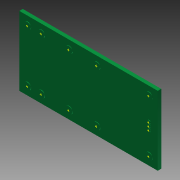
# Autodesk Inventor part: PDU
Saved by Autodesk Inventor 2011 SP1 (Build 150282100, 282)
## iProperties
Created: 2011-06-14
Part Number: PDU
Document SubType Name: Modeling
Designer: Andrew G. Meyer
Mass: 3.22222 g
Surface Area: 43.638 cm^2
Volume: 3.22222 cm^3
Density: 1 g/cm^3
GlobalPropertyList: <PropertyList/>
Author: Andrew G. Meyer
Autodesk Inventor part; units mm, degrees
ref_plane "YZ Plane" through (0, 0, 0) normal (1, 0, 0) x (0, 1, 0)
ref_plane "XZ Plane" through (0, 0, 0) normal (0, 1, 0) x (-1, 0, 0)
ref_plane "XY Plane" through (0, 0, 0) normal (0, 0, 1) x (1, 0, 0)
sketch "Sketch1" plane through (0, 0, 0) normal (0, 0, 1) x (1, 0, 0)
  line L0 (-25.8084, 16.7799) -> (37.6916, 16.7799)
  line L1 (37.6916, 16.7799) -> (37.6916, -14.9701)
  line L2 (37.6916, -14.9701) -> (-25.8084, -14.9701)
  line L3 (-25.8084, -14.9701) -> (-25.8084, 16.7799)
  point P0 (0, 0)
  dimension "d0" = 31.75
  dimension "d1" = 63.5
  constraints: 8 end point, 2 parallel, 1 horizontal, 1 perpendicular
  measures "d0" distance of L2.end L0.start
  measures "d1" distance of L0.start L0.end
extrude "Extrusion1" add sketch "Sketch1" along normal blind 1.5875
sketch "Sketch2" plane through (0, 0, 1.5875) normal (0, 0, 1) x (1, 0, 0)
  line L0 (37.6916, 16.7799) -> (37.6916, -14.9701) projected
  line L1 (-25.8084, 16.7799) -> (37.6916, 16.7799) projected
  line L2 (-25.8084, -14.9701) -> (-25.8084, 16.7799) projected
  line L3 (37.6916, -14.9701) -> (-25.8084, -14.9701) projected
  circle A0 centre (33.813, 12.9013) radius 1.5875
  circle A1 centre (33.813, -11.0915) radius 1.5875
  circle A2 centre (33.813, 2.4924) radius 0.7937
  circle A3 centre (33.813, 0.9049) radius 0.7937
  circle A4 centre (33.813, -0.6826) radius 0.7937
  line L4 (33.813, -14.9701) -> (33.813, 16.7799) construction
  line L5 (33.813, 2.4924) -> (33.813, 0.9049) construction
  line L6 (33.813, 0.9049) -> (33.813, -0.6826) construction
  line L7 (33.813, 12.9013) -> (33.813, 2.4924) construction
  line L8 (33.813, -11.0915) -> (33.813, -0.6826) construction
  circle A5 centre (-21.9298, 12.9013) radius 1.5875
  circle A6 centre (-21.9298, -11.0915) radius 1.5875
  line L9 (-21.9298, 16.7799) -> (-21.9298, -14.9701) construction
  line L10 (-25.8084, -11.0915) -> (37.6916, -11.0915) construction
  circle A7 centre (-15.5798, 12.9013) radius 1.5875
  circle A8 centre (-15.5798, -11.0915) radius 1.5875
  circle A9 centre (-2.8798, 12.9013) radius 1.5875
  circle A10 centre (-2.8798, -11.0915) radius 1.5875
  circle A11 centre (9.8202, 12.9013) radius 1.5875
  circle A12 centre (9.8202, -11.0915) radius 1.5875
  point P0 (0, 0)
  dimension "d4" = 3.8786
  dimension "d5" = 3.8786
  dimension "d6" = 3.8786
  dimension "d7" = 3.175
  dimension "d8" = 1.5875
  dimension "d9" = 3.175
  dimension "d10" = 3.8786
  dimension "d11" = 3.8786
  dimension "d14" = 6.35
  dimension "d21" = 12.7
  dimension "d28" = 12.7
  constraints: 14 end point, 14 point on line, 13 centre point, 6 collinear, 5 equal radius, 3 horizontal, 3 perpendicular, 1 midpoint, 12 other
  measures "d4" distance from line of L7.start L1
  measures "d5" distance from line of L3 L8.start
  measures "d6" distance from line of L0 L8.start
  measures "d7" diameter of A0
  measures "d8" diameter of A2
  measures "d9" diameter of A5
  measures "d10" distance from line of L2 A5.centre
  measures "d11" distance from line of L1 A5.centre
  measures "d14" distance of A5.centre A7.centre
  measures "d21" distance of A7.centre A9.centre
  measures "d28" distance of A9.centre A11.centre
extrude "Extrusion2" add sketch "Sketch2" along normal blind 0.254 contours A0 | A1 | A2 | A4 | A3 | A5 | A6 | A7 | A8 | A9 | A10 | A11 | A12
sketch "Sketch3" plane through (33.813, 12.9013, 1.8415) normal (0, 0, 1) x (1, 0, 0)
  circle A0 centre (0, 0) radius 1.5875 construction
sketch "Sketch4" plane through (33.813, -11.0915, 1.8415) normal (0, 0, 1) x (1, 0, 0)
  circle A0 centre (0, 0) radius 1.5875 construction
sketch "Sketch5" plane through (9.8202, 12.9013, 1.8415) normal (0, 0, 1) x (1, 0, 0)
  circle A0 centre (0, 0) radius 1.5875 construction
sketch "Sketch6" plane through (9.8202, -11.0915, 1.8415) normal (0, 0, 1) x (1, 0, 0)
  circle A0 centre (0, 0) radius 1.5875 construction
sketch "Sketch7" plane through (-2.8798, 12.9013, 1.8415) normal (0, 0, 1) x (1, 0, 0)
  circle A0 centre (0, 0) radius 1.5875 construction
sketch "Sketch8" plane through (-2.8798, -11.0915, 1.8415) normal (0, 0, 1) x (1, 0, 0)
  circle A0 centre (0, 0) radius 1.5875 construction
sketch "Sketch9" plane through (-15.5798, 12.9013, 1.8415) normal (0, 0, 1) x (1, 0, 0)
  circle A0 centre (0, 0) radius 1.5875 construction
sketch "Sketch10" plane through (-15.5798, -11.0915, 1.8415) normal (0, 0, 1) x (1, 0, 0)
  circle A0 centre (0, 0) radius 1.5875 construction
sketch "Sketch11" plane through (-21.9298, 12.9013, 1.8415) normal (0, 0, 1) x (1, 0, 0)
  circle A0 centre (0, 0) radius 1.5875 construction
sketch "Sketch12" plane through (-21.9298, -11.0915, 1.8415) normal (0, 0, 1) x (1, 0, 0)
  circle A0 centre (0, 0) radius 1.5875 construction
sketch "Sketch13" plane through (33.813, -0.6826, 1.8415) normal (0, 0, 1) x (1, 0, 0)
  circle A0 centre (0, 0) radius 0.7937 construction
  point P0 (0, 0.7937)
  constraints: 1 vertical alignment
sketch "Sketch14" plane through (0, 0, 1.8415) normal (0, 0, 1) x (1, 0, 0)
  arc A0 (33.813, 0.1112) -> (33.813, 1.6987) centre (33.813, 0.9049) ccw construction
sketch "Sketch15" plane through (33.813, 2.4924, 1.8415) normal (0, 0, 1) x (1, 0, 0)
  circle A0 centre (0, 0) radius 0.7937 construction
  point P0 (0, -0.7937)
  constraints: 1 vertical alignment
equation "\"d5\" = d4"
equation "\"d6\" = d4"
equation "\"d10\" = d4"
equation "\"d11\" = d4"
body "Solid1"
